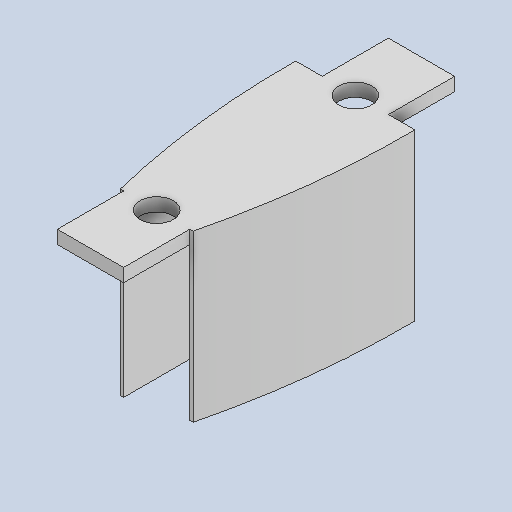
# Autodesk Inventor part: squeezer
Saved by Autodesk Inventor 2025 (Build 290162000, 162)
## iProperties
Created: 2025-08-15
Part Number: squeezer
Material: Generic
Document SubType Name: Modeling
Designer: Pravoslav
Density: 1 g/cm^3
Appearance: Default
Author: Pravoslav
Autodesk Inventor part; units mm, degrees
note: some values were not read from the file. Chosen so that the rebuilt part matches the saved one: second side of "Extrusion3".
ref_plane "YZ Plane" through (0, 0, 0) normal (1, 0, 0) x (0, 1, 0)
ref_plane "XZ Plane" through (0, 0, 0) normal (0, 1, 0) x (-1, 0, 0)
ref_plane "XY Plane" through (0, 0, 0) normal (0, 0, 1) x (1, 0, 0)
sketch "Sketch1" plane through (0, 0, 0) normal (0, 1, 0) x (-1, 0, 0)
  line L0 (5, 25) -> (-5, 25)
  line L1 (-5, 25) -> (-5, -25)
  line L2 (-5, -25) -> (5, -25)
  line L3 (5, -25) -> (5, 25)
  line L4 (5, 25) -> (-5, -25) construction
  line L5 (-5, 25) -> (5, -25) construction
  circle A0 centre (0, 15) radius 2.5
  circle A1 centre (0, -15) radius 2.5
  point P0 (0, 0)
  point P1 (0, 25)
  dimension "d0" = 10
  dimension "d1" = 50
  dimension "d2" = 5
  dimension "d3" = 5
  dimension "d4" = 30
  dimension "d5" = 10
  dimension "d6" = 5
  dimension "d7" = 5
  constraints: 12 end point, 3 midpoint, 2 centre point, 2 parallel, 1 horizontal, 1 perpendicular
  measures "d0" distance of L2.end L1.end
  measures "d1" distance of L1.end L0.end
  measures "d2" diameter of A0
  measures "d3" diameter of A1
  measures "d4" distance of A1.centre A0.centre
  measures "d5" distance of point (0, 25) A0.centre
  measures "d6" distance from line of L1 A0.centre
  measures "d7" distance from line of L1 A1.centre
extrude "Extrusion1" add sketch "Sketch1" along normal blind 2
sketch "Sketch2" plane through (0, 0, 0) normal (0, -1, 0) x (1, 0, 0)
  line L0 (-5, -15) -> (-9, -15)
  line L1 (-5, 15) -> (-5.5, 15)
  circle A0 centre (0, -15) radius 2.5 projected
  circle A1 centre (0, 15) radius 2.5 projected
  arc A2 (-5.5, 15) -> (-9, -15) centre (110.994, -13.7951) ccw
  line L2 (-5, -15) -> (-5, 15)
  line L3 (-5, -25) -> (-5, 25) projected
  point P0 (0, 0)
  point P1 (-4, -14.9499)
  point P2 (-3, -15)
  dimension "d10" = 0
  dimension "d11" = 0
  dimension "d12" = 4
  dimension "d13" = 0.5
  dimension "d14" = 120
  dimension "d15" = 0
  dimension "d16" = 0
  dimension "d17" = 0
  constraints: 6 end point, 2 horizontal, 2 point on circle, 1 centre point, 1 vertical
  measures "d10" distance from line of A0.centre L0
  measures "d11" distance from line of A1.centre L1
  measures "d12" distance of L0.start L0.end
  measures "d13" distance of L1.start L1.end
  measures "d14" radius of A2
  measures "d15" distance of L0.start L2.start
  measures "d16" distance between parallel lines of L3 L2
  measures "d17" distance of L2.end L1.start
extrude "Extrusion2" add sketch "Sketch2" along normal blind 25 and the other way blind 2 contours L0 A2 L1 L2
sketch "Sketch3" plane through (0, 2, 0) normal (0, 1, 0) x (1, 0, 0)
  line L0 (5, -25) -> (5, 25) projected
  line L1 (5, 15) -> (9, 15)
  line L2 (5, -15) -> (5.5, -15)
  line L3 (5, -15) -> (5, 15)
  circle A0 centre (0, 15) radius 2.5 projected
  circle A1 centre (0, -15) radius 2.5 projected
  arc A2 (5.5, -15) -> (9, 15) centre (-110.994, 13.7951) ccw
  point P0 (0, 0)
  dimension "d22" = 0
  dimension "d23" = 0
  dimension "d24" = 0.5
  dimension "d25" = 4
  dimension "d26" = 120
  constraints: 6 end point, 2 horizontal, 2 point on circle, 2 point on line, 1 centre point, 1 collinear
  measures "d22" distance from line of A0.centre L1
  measures "d23" distance from line of A1.centre L2
  measures "d24" distance of L2.start L2.end
  measures "d25" distance of L1.start L1.end
  measures "d26" radius of A2
extrude "Extrusion3" add sketch "Sketch3" against normal blind 25 contours L0 L1 A2 L2
body "Solid1"
